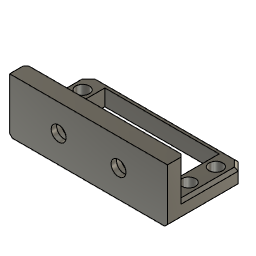
servo_holder (Autodesk Fusion 360 design; units mm, degrees)
Autodesk Fusion 360 part; units mm, degrees
sketch "Sketch1" plane through (0, 0, 0) normal (0, 0, 1) x (1, 0, 0) in component "Servohalterung"
  line L0 (0, 0) -> (58, 0)
  line L1 (58, 0) -> (58, 29)
  line L2 (58, 29) -> (0, 29)
  line L3 (0, 29) -> (0, 0)
  line L4 (8, 27) -> (50, 27)
  line L5 (50, 27) -> (50, 6)
  line L6 (50, 6) -> (8, 6)
  line L7 (8, 6) -> (8, 27)
  dimension "d22" = 8
  dimension "d23" = 8
  dimension "d24" = 42
  dimension "d25" = 2
  dimension "d26" = 6
  dimension "d27" = 21
  constraint horizontal L0
  constraint vertical L1
  constraint horizontal L2
  constraint vertical L3
  constraint coincident L0.start L3.end
  constraint horizontal L4
  constraint vertical L5
  constraint horizontal L6
  constraint vertical L7
  measures "d22" distance of L0.start L7
  measures "d23" distance of L1 L5
  measures "d24" distance of L4.start L4.end
  measures "d25" distance of L2 L4
  measures "d26" distance of L0 L6
  measures "d27" distance of L4.end L5.end
extrude "Extrude1" add sketch "Sketch1" along normal blind 6 in component "Servohalterung"
sketch "Sketch2" plane through (0, 0, 6) normal (0, 0, 1) x (-1, 0, 0) in component "Servohalterung"
  line L0 (-50, -6) -> (-8, -6)
  line L1 (-8, -6) -> (-8, -27)
  line L2 (-8, -27) -> (-50, -27)
  line L3 (-50, -27) -> (-50, -6)
  line L4 (0, -29) -> (0, 0)
  line L5 (0, 0) -> (-58, 0)
  line L6 (-58, 0) -> (-58, -29)
  line L7 (-58, -29) -> (0, -29)
  line L8 (0, 0) -> (-58, 0)
  line L9 (-58, 0) -> (-58, -6)
  line L10 (-58, -6) -> (0, -6)
  line L11 (0, -6) -> (0, 0)
  line L12 (-50, -6) -> (-8, -6)
  constraint horizontal L8
  constraint vertical L9
  constraint horizontal L10
  constraint vertical L11
  constraint coincident L6 L9.end
  constraint coincident L4.end L5.start
  constraint collinear L10 L12
extrude "Extrude2" add sketch "Sketch2" along normal blind 14 contours L0 L4 L5 L6 L8 L9 L10 L11 L12 in component "Servohalterung"
sketch "Sketch3" plane through (0, 6, 0) normal (0, 1, 0) x (-1, 0, 0) in component "Servohalterung"
  line L0 (-8, 0) -> (-8, 6)
  line L1 (-8, 6) -> (0, 6)
  line L2 (0, 6) -> (0, 20)
  line L3 (0, 20) -> (-58, 20)
  line L4 (-58, 20) -> (-58, 6)
  line L5 (-58, 6) -> (-50, 6)
  line L6 (-50, 6) -> (-50, 0)
  line L7 (-50, 0) -> (-8, 0)
  circle A0 centre (-40, 10) radius 6
  line L8 (-29, 0) -> (-29, 20)
  circle A1 centre (-18, 10) radius 6
  dimension "d34" = 12
  dimension "d38" = 10
  dimension "d64" = 10
  constraint midpoint L3 L8.end
  constraint symmetric A0 L8 A1
  constraint midpoint L7 L8.start
  measures "d34" diameter of A0
  measures "d38" distance of L6 A0.centre
  measures "d64" distance of L3 A0.centre
extrude "Extrude3" cut sketch "Sketch3" against normal blind 4 contours A0 | A1 in component "Servohalterung"
sketch "Sketch4" plane through (0, 2, 0) normal (0, 1, 0) x (-1, 0, 0) in component "Servohalterung"
  circle A0 centre (-40, 10) radius 6
  circle A1 centre (-40, 10) radius 2.75
  line L0 (-28.3646, -4) -> (-28.3646, 24)
  circle A2 centre (-18, 10) radius 2.75
  circle A3 centre (-18, 10) radius 6
  line L1 (-58, 20) -> (0, 20)
  dimension "d42" = 5.5
  dimension "d43" = 5.5
  constraint concentric A0 A1
  constraint concentric A2 A3
  measures "d42" diameter of A1
  measures "d43" diameter of A2
extrude "Extrude4" cut sketch "Sketch4" against normal up to surface (2 mm away) contours A1 | A2 in component "Servohalterung"
sketch "Sketch5" plane through (0, 0, 6) normal (0, 0, 1) x (-1, 0, 0) in component "Servohalterung"
  line L0 (0, -6) -> (-8, -6)
  line L1 (-8, -6) -> (-8, -27)
  line L2 (-8, -27) -> (-50, -27)
  line L3 (-50, -27) -> (-50, -6)
  line L4 (-50, -6) -> (-58, -6)
  line L5 (-58, -6) -> (-58, -29)
  line L6 (-58, -29) -> (0, -29)
  line L7 (0, -29) -> (0, -6)
  circle A0 centre (-4.5, -22.3) radius 2.5
  circle A1 centre (-4.5, -12.3) radius 2.5
  circle A2 centre (-53.5, -22.3) radius 2.5
  circle A3 centre (-53.5, -12.3) radius 2.5
  dimension "d46" = 5
  dimension "d48" = 2.2
  dimension "d49" = 1
  dimension "d50" = 5
  dimension "d51" = 5
  dimension "d52" = 5
  dimension "d53" = 5
  dimension "d54" = 5
  dimension "d57" = 1
  constraint vertical A0.centre A1.centre
  constraint vertical A3.centre A2.centre
  constraint horizontal A0.centre A2.centre
  measures "d46" diameter of A0
  measures "d48" distance of L2 A0
  measures "d49" distance of L1 A0
  measures "d50" diameter of A1
  measures "d51" distance of A0 A1
  measures "d52" diameter of A2
  measures "d53" diameter of A3
  measures "d54" distance of A2 A3
  measures "d57" distance of L3 A2
extrude "Extrude5" cut sketch "Sketch5" against normal up to surface (6 mm away) contours A0 | A1 | A2 | A3 in component "Servohalterung"
chamfer "Chamfer3" distance 3 angle 45 2 edges at (58, 29, 3) (0, 29, 3) in component "Servohalterung"
chamfer "Chamfer1" distance 1 angle 45 12 edges at (58, 13, 0) (58, 16, 6) (29, 29, 6) (29, 29, 0) (0, 13, 0) (0, 16, 6) (1.5, 27.5, 0) (1.5, 27.5, 6) (56.5, 27.5, 0) (56.5, 27.5, 6) (0, 6, 13) (58, 6, 13) in component "Servohalterung"
component "Servohalterung" placed x (1, 0, 0) y (0, 1, 0) z (0, 0, 1) at (0, 0, 0)
